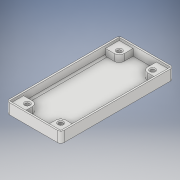
# Autodesk Inventor part: photocouplerboard_hf_base_sa_1
Saved by Autodesk Inventor 2019 (Build 230136000, 136)
## iProperties
Created: 2019-02-28
Part Number: photocouplerboard_hf_base_sa_1
Material: ABS プラスチック
Document SubType Name: Modeling
Designer: shun
Density: 1.06 g/cm^3
Appearance: 滑らか - 白
Author: shun
Autodesk Inventor part; units mm, degrees
ref_plane "YZ Plane" through (0, 0, 0) normal (1, 0, 0) x (0, 1, 0)
ref_plane "XZ Plane" through (0, 0, 0) normal (0, 1, 0) x (-1, 0, 0)
ref_plane "XY Plane" through (0, 0, 0) normal (0, 0, 1) x (1, 0, 0)
sketch "スケッチ1" plane through (0, 0, 0) normal (0, 1, 0) x (-1, 0, 0)
  line L0 (15, 32.5) -> (-15, 32.5) construction
  line L1 (-15, 32.5) -> (-15, -32.5) construction
  line L2 (-15, -32.5) -> (15, -32.5) construction
  line L3 (15, -32.5) -> (15, 32.5) construction
  line L4 (15, 32.5) -> (-15, -32.5) construction
  line L5 (-15, 32.5) -> (15, -32.5) construction
  line L6 (15.3, 32.8) -> (-15.3, 32.8)
  line L7 (-15.3, 32.8) -> (-15.3, -32.8)
  line L8 (-15.3, -32.8) -> (15.3, -32.8)
  line L9 (15.3, -32.8) -> (15.3, 32.8)
  line L10 (16.3, 33.8) -> (-16.3, 33.8)
  line L11 (-16.3, 33.8) -> (-16.3, -33.8)
  line L12 (-16.3, -33.8) -> (16.3, -33.8)
  line L13 (16.3, -33.8) -> (16.3, 33.8)
  line L14 (-10, 27.5) -> (10, 27.5) construction
  line L15 (10, 27.5) -> (10, -27.5) construction
  line L16 (10, -27.5) -> (-10, -27.5) construction
  line L17 (-10, -27.5) -> (-10, 27.5) construction
  line L18 (7, 32.8) -> (7, 27.5)
  arc A0 (7, 27.5) -> (10, 24.5) centre (10, 27.5) ccw
  line L19 (10, 24.5) -> (15.3, 24.5)
  line L20 (0, 0) -> (0, 32.8)
  line L21 (0, 32.8) -> (0, 33.8)
  line L22 (0, 0) -> (15.3, 0)
  line L23 (15.3, 0) -> (16.3, 0)
  dimension "d0" = 30
  dimension "d1" = 65
  dimension "d2" = 0.3
  dimension "d3" = 1
  dimension "d4" = 5
  dimension "d5" = 3
  constraints: 48 end point, 8 parallel, 6 midpoint, 6 perpendicular, 5 coincident, 4 point on line, 2 point on circle, 1 centre point, 1 horizontal, 9 other
  measures "d0" distance of L2.end L1.end
  measures "d1" distance of L1.end L0.end
  measures "d2" distance between parallel lines of L3 L9
  measures "d3" distance between parallel lines of L9 L13
  measures "d4" distance between parallel lines of L0 L14
  measures "d5" distance from line of L18 point (10, 27.5)
extrude "押し出し1" add sketch "スケッチ1" against normal blind 0.8 contours L9 L19 A0 L18 L6 | L6 L21 L10 L13 L23 L9 | L18 A0 L19 L9 L22 L20 L6
extrude "押し出し2" add sketch "スケッチ1" along normal blind 4 contours L9 L19 A0 L18 L6
extrude "押し出し3" add sketch "スケッチ1" along normal blind 1.5 and the other way blind 4 from surface at 4 contours L6 L21 L10 L13 L23 L9
hole "穴1" at (10, 0, 27.5) at (-10, 0, 27.5) at (-10, 0, -27.5) at (10, 0, -27.5) direction (0, -1, 0) diameter 2.5 end through all both
fillet "フィレット1" radius 0.5 1 edges at (-10, 4, 26.25)
mirror "ミラー1" about plane through (-16.3, 0, 0) normal (0, 0, -1) of "フィレット1", "穴1", "押し出し3", "押し出し2", "押し出し1"
mirror "ミラー2" about plane through (0, 0, 32.8) normal (1, 0, 0) of "フィレット1", "穴1", "押し出し3", "押し出し2", "押し出し1", "ミラー1"
fillet "フィレット2" radius 1 2 edges at (-15.3, 0, 0) (0, 0, 32.8)
fillet "フィレット3" radius 2 4 edges at (16.3, 2.35, 33.8) (-16.3, 2.35, 33.8) (-16.3, 2.35, -33.8) (16.3, 2.35, -33.8)
